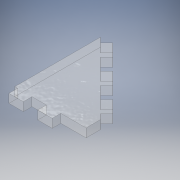
# Autodesk Inventor part: phone_holder_slider_side
Saved by Autodesk Inventor 2019 (Build 230136000, 136)
## iProperties
Created: 2019-02-17
Part Number: phone_holder_slider_side
Material: Acrylic, Clear
Document SubType Name: Modeling
Designer: suchanek
Density: 1.19 g/cm^3
Appearance: Transparent - Clear
Author: suchanek
Autodesk Inventor part; units mm, degrees
ref_plane "YZ Plane" through (0, 0, 0) normal (1, 0, 0) x (0, 1, 0)
ref_plane "XZ Plane" through (0, 0, 0) normal (0, 1, 0) x (-1, 0, 0)
ref_plane "XY Plane" through (0, 0, 0) normal (0, 0, 1) x (1, 0, 0)
sketch "Sketch2" plane through (0, 0, 0) normal (0, 1, 0) x (-1, 0, 0)
  line L0 (-24.7487, 5) -> (24.7487, 5)
  line L1 (24.7487, 5) -> (24.7487, -5)
  line L2 (24.7487, -5) -> (-24.7487, -5)
  line L3 (-24.7487, -5) -> (-24.7487, 5)
  line L4 (-24.7487, 5) -> (24.7487, -5) construction
  line L5 (24.7487, 5) -> (-24.7487, -5) construction
  line L6 (22.7487, 11) -> (12.7487, 11)
  line L7 (12.7487, 11) -> (12.7487, 5)
  line L8 (12.7487, 5) -> (22.7487, 5)
  line L9 (22.7487, 5) -> (22.7487, 11)
  line L10 (-24.7487, -5) -> (24.7487, -54.4975)
  line L11 (-24.7487, -5) -> (45.2513, -5) construction
  line L12 (24.7487, -54.4975) -> (24.7487, -5)
  line L13 (21.2132, -50.9619) -> (12.7279, -42.4767)
  line L14 (12.7279, -42.4767) -> (8.4853, -46.7193)
  line L15 (8.4853, -46.7193) -> (16.9706, -55.2046)
  line L16 (16.9706, -55.2046) -> (21.2132, -50.9619)
  line L17 (4.2426, -33.9914) -> (-4.2426, -25.5061)
  line L18 (0, -38.234) -> (4.2426, -33.9914)
  line L19 (-8.4853, -29.7487) -> (0, -38.234)
  line L20 (-4.2426, -25.5061) -> (-8.4853, -29.7487)
  line L21 (-12.7279, -17.0208) -> (-21.2132, -8.5355)
  line L22 (-16.9706, -21.2635) -> (-12.7279, -17.0208)
  line L23 (-25.4558, -12.7782) -> (-16.9706, -21.2635)
  line L24 (-21.2132, -8.5355) -> (-25.4558, -12.7782)
  line L25 (2.7487, 5) -> (-7.2513, 5)
  line L26 (-7.2513, 5) -> (-7.2513, 11)
  line L27 (-7.2513, 11) -> (2.7487, 11)
  line L28 (2.7487, 11) -> (2.7487, 5)
  point P0 (0, 0)
  dimension "d9" = 10
  dimension "d19" = 10
  dimension "d20" = 6
  dimension "d21" = 2
  dimension "d40" = 70
  dimension "d41" = 45
  dimension "d42" = 6
  dimension "d45" = 24
  dimension "d50" = 5
  dimension "d51" = 12
  dimension "d52" = 10
  dimension "d53" = 6
  dimension "d54" = 10
  constraints: 58 end point, 8 parallel, 4 horizontal, 4 perpendicular, 3 point on line, 2 midpoint, 1 collinear, 1 equal length, 1 vertical, 17 other
  measures "d9" distance of L0.end L1.end
  measures "d19" distance of L8.end L7.end
  measures "d20" distance of L7.end L6.end
  measures "d21" distance between parallel lines of L1 L9
  measures "d40" distance of L2.end L10.end
  measures "d41" angle of L10 L11
  measures "d42" distance of L14.end L13.end
  measures "d45" distance of L13.end L17.end
  measures "d50" distance from line of L10.end L16
  measures "d51" distance of L14.end L15.end
  measures "d52" distance of L26.end L27.end
  measures "d53" distance of L25.end L26.end
  measures "d54" distance between parallel lines of L28 L7
extrude "Extrusion2" add sketch "Sketch2" along normal blind 6
body "Solid2"
